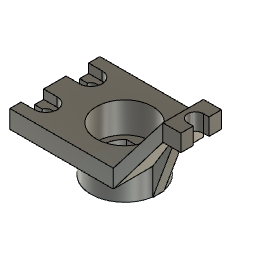
drawing_13 v1 (Autodesk Fusion 360 design; units mm, degrees)
Autodesk Fusion 360 part; units mm, degrees
sketch "Sketch1" plane through (0, 0, 0) normal (0, 0, 1) x (1, 0, 0)
  circle A0 centre (0, 0) radius 30
  constraint coincident A0.centre origin
extrude "Extrude1" add sketch "Sketch1" along normal blind 24 makes body 1
sketch "Sketch2" plane through (0, 0, 24) normal (0, 0, 1) x (-1, 0, 0)
  circle A0 centre (0, 0) radius 30
  line L0 (-30, 0) -> (-30, -40)
  line L1 (-30, -40) -> (-30, 0)
  line L2 (-30, 0) -> (-30, 40)
  line L3 (0, -40) -> (62, -40)
  line L4 (62, -40) -> (-30, -40)
  line L5 (-30, -40) -> (-30, 40)
  line L6 (-30, 40) -> (62, 40)
  line L7 (62, 40) -> (62, -40)
  constraint coincident A0.centre origin
  constraint coincident A0 L0.start
  constraint tangent A0 L1
  constraint perpendicular L0 L3
  constraint horizontal L4
  constraint vertical L5
  constraint horizontal L6
  constraint vertical L7
extrude "Extrude2" add sketch "Sketch2" along normal blind 16 contours A0 | L0 L1 L2 L3 L4 L5 L6 L7 bodies 1
sketch "Sketch3" plane through (0, 0, 40) normal (0, 0, 1) x (-1, 0, 0)
  line L0 (62, 40) -> (-30, 40)
  line L1 (-30, 40) -> (-30, -40)
  line L2 (-30, -40) -> (62, -40)
  line L3 (62, -40) -> (62, 40)
  line L4 (62, 0) -> (62, -20)
  line L5 (62, 0) -> (62, 20)
  line L6 (55.1235, 22) -> (62, 22)
  line L7 (62, 22) -> (62, 18)
  line L8 (62, 18) -> (55.1235, 18)
  line L9 (55.1235, -18) -> (62, -18)
  line L10 (62, -18) -> (62, -22)
  line L11 (62, -22) -> (55.1235, -22)
  arc A0 (59.798, -18) -> (59.798, -22) centre (50, -20) ccw
  arc A1 (55.1235, -18) -> (55.1235, -22) centre (50, -20) ccw
  arc A2 (59.798, 22) -> (59.798, 18) centre (50, 20) ccw
  arc A3 (55.1235, 22) -> (55.1235, 18) centre (50, 20) ccw
  point P0 (62, 0)
  constraint midpoint L3 P0
  constraint coincident P0 L4.start
  constraint parallel L3 L4
  constraint parallel L3 L5
  constraint concentric A0 A1
  constraint concentric A2 A3
  constraint horizontal L6
  constraint vertical L7
  constraint horizontal L8
  constraint coincident L3 L7.end
  constraint horizontal L9
  constraint vertical L10
  constraint horizontal L11
  constraint coincident L11 A0.end
  constraint coincident L9 A0.start
  constraint coincident L8 A2.end
  constraint coincident L6 A2.start
extrude "Extrude3" cut sketch "Sketch3" against normal blind 123 contours L3 L5 L6 L7 L8 A3 | L3 L4 L9 L10 L11 A1 bodies 1
sketch "Sketch4" plane through (0, 0, 40) normal (0, 0, 1) x (-1, 0, 0)
  line L0 (55.1235, 22) -> (62, 22)
  line L1 (62, 22) -> (62, 40)
  line L2 (62, 40) -> (-30, 40)
  line L3 (-30, 40) -> (-30, -40)
  line L4 (-30, -40) -> (62, -40)
  line L5 (62, -40) -> (62, -22)
  line L6 (62, -22) -> (55.1235, -22)
  arc A0 (55.1235, -18) -> (55.1235, -22) centre (50, -20) ccw
  line L7 (55.1235, -18) -> (62, -18)
  line L8 (62, -18) -> (62, 18)
  line L9 (62, 18) -> (55.1235, 18)
  arc A1 (55.1235, 22) -> (55.1235, 18) centre (50, 20) ccw
  circle A2 centre (50, -20) radius 10
  circle A3 centre (50, 20) radius 10
  line L10 (50, -30) -> (50, -10)
  line L11 (50, 30) -> (50, 10)
  line L12 (50, -30) -> (62, -30)
  line L13 (50, -10) -> (62, -10)
  line L14 (50, 10) -> (62, 10)
  line L15 (50, 30) -> (62, 30)
  dimension "d25" = 20
  dimension "d26" = 20
  constraint concentric A0 A2
  constraint concentric A1 A3
  constraint coincident A2 L10.start
  constraint coincident A2 L10.end
  constraint parallel L5 L10
  constraint coincident A3 L11.start
  constraint coincident A3 L11.end
  constraint parallel L10 L11
  constraint coincident L5 L12.end
  constraint tangent A2 L12
  constraint perpendicular L5 L12
  constraint coincident L8 L13.end
  constraint tangent A2 L13
  constraint coincident L8 L14.end
  constraint tangent A3 L14
  constraint perpendicular L8 L14
  constraint coincident L1 L15.end
  constraint tangent A3 L15
  measures "d25" diameter of A2
  measures "d26" diameter of A3
extrude "Extrude4" cut sketch "Sketch4" against normal blind 8 contours L0 A1 A3 L11 | L0 L1 A3 L15 | A1 A3 L11 | L9 A1 A3 L11 | L8 L9 A3 L14 | L7 L8 A2 L13 | A0 A2 L10 | A0 L7 A2 L10 | L6 A0 A2 L10 | L5 L6 A2 L12 bodies 1
sketch "Sketch5" plane through (0, -40, 0) normal (0, -1, 0) x (1, 0, 0)
  line L0 (-62, 24) -> (30, 24)
  line L1 (30, 24) -> (30, 40)
  line L2 (30, 40) -> (-62, 40)
  line L3 (-62, 40) -> (-62, 24)
  line L4 (52, 55) -> (52, 70)
  line L5 (52, 70) -> (52, 55)
  line L6 (30, 40) -> (52, 70)
  line L7 (30, 24) -> (52, 55)
  constraint coincident L1.end L2.start
  constraint parallel L4 L5
  constraint coincident L0.end L1.start
sketch "Sketch6" plane through (0, 40, 0) normal (0, 1, 0) x (-1, 0, 0)
  line L0 (-30, 24) -> (62, 24)
  line L1 (62, 24) -> (62, 40)
  line L2 (62, 40) -> (-30, 40)
  line L3 (-30, 40) -> (-30, 24)
  line L4 (62, 24) -> (-52, 24)
  line L5 (-52, 24) -> (-52, 26)
  line L6 (-52, 26) -> (-30, 26)
  line L7 (-30, 24) -> (-30, 26)
  dimension "d34" = 114
  dimension "d35" = 2
  constraint coincident L0.end L1.start
  constraint perpendicular L1 L4
  constraint perpendicular L4 L5
  constraint coincident L3 L6.end
  constraint perpendicular L3 L6
  constraint coincident L0.start L3.end
  measures "d34" distance of L0.end L4.end
  measures "d35" distance of L4.end L5.end
ref_plane "WorkPlane3" through (0, 0, 75) normal (0, 0, -1) x (-1, 0, 0)
sketch "Sketch23" plane through (0, 0, 75) normal (0, 0, -1) x (1, 0, 0)
  line L0 (-62, -30) -> (-50, -30) construction
  arc A0 (-50, -30) -> (-50, -10) centre (-50, -20) ccw construction
  line L1 (-50, -10) -> (-62, -10) construction
  line L2 (-62, -10) -> (-62, 10) construction
  line L3 (-62, 10) -> (-50, 10) construction
  arc A1 (-50, 10) -> (-50, 30) centre (-50, 20) ccw construction
  line L4 (-50, 30) -> (-62, 30) construction
  line L5 (-62, 30) -> (-62, 40) construction
  line L6 (-62, 40) -> (30, 40) construction
  line L7 (30, 40) -> (30, -40) construction
  line L8 (30, -40) -> (-62, -40) construction
  line L9 (-62, -40) -> (-62, -30) construction
  line L10 (-62, 0) -> (68, 0) construction
  line L11 (68, 0) -> (52, 0) construction
  line L12 (52, 0) -> (52, -18) construction
  line L13 (52, -18) -> (52, 18) construction
  line L14 (68, -18) -> (52, -18)
  line L15 (52, -18) -> (52, 18)
  line L16 (52, 18) -> (68, 18)
  line L17 (68, 18) -> (68, -18)
  line L18 (68, -18) -> (52, 18) construction
  line L19 (52, -18) -> (68, 18) construction
  circle A2 centre (0, 0) radius 30 construction
  line L20 (0, 0) -> (63, 0) construction
  line L21 (63, -7) -> (77.3975, -7)
  arc A3 (77.3975, -7) -> (77.3975, 7) centre (77.3975, 0) ccw
  line L22 (77.3975, 7) -> (63, 7)
  arc A4 (63, 7) -> (63, -7) centre (63, 0) ccw
  line L23 (63, 0) -> (77.3975, 0) construction
  point P0 (60, 0)
  dimension "d68" = 130
  dimension "d69" = 16
  dimension "d72" = 16
  dimension "d73" = 36
  dimension "d74" = 63
  dimension "d75" = 14
  constraint midpoint L2 L10.start
  constraint perpendicular L2 L10
  constraint coincident L10 L11.end
  constraint perpendicular L11 L12
  constraint perpendicular L10 L13
  constraint horizontal L14
  constraint perpendicular L14 L15
  constraint parallel L14 L16
  constraint parallel L15 L17
  constraint coincident L18 P0
  constraint coincident L19 P0
  constraint midpoint L11 P0
  constraint coincident A2.centre L20.start
  constraint parallel L10 L20
  constraint tangent L21 A3
  constraint tangent A3 L22
  constraint parallel L21 L22
  constraint tangent L22 A4
  constraint tangent L21 A4
  constraint perpendicular L17 L23
  constraint coincident L20.end A4.centre
  measures "d68" distance of L10.start L10.end
  measures "d69" distance of L10.end L11.end
  measures "d72" distance of L13.end L16.end
  measures "d73" distance of L12.end L13.end
  measures "d74" distance of A2.centre L20.end
  measures "d75" diameter of A3
extrude "Extrude15" add sketch "Sketch23" along normal blind 15 separate body contours L14 L15 L16 L17 L21 L22 A4 makes body 2
loft "Loft1" add section 1 face at (52, 6, 70) section 2 face at (30, 0, 34.6667) on bodies 1 2 bodies 2 1
sketch "Sketch24" plane through (0, 0, 0) normal (0, 1, 0) x (1, 0, 0)
  line L0 (52, -75) -> (30, -40)
  line L1 (52, -60) -> (30, -24)
  line L2 (-62, -40) -> (30, -40)
  line L3 (-62, -24) -> (-62, -40)
  line L4 (-30, -24) -> (-62, -24)
  line L5 (-30, 0) -> (30, 0)
  line L6 (52, -75) -> (68, -75)
  line L7 (68, -60) -> (52, -60)
  line L8 (68, -75) -> (68, -60)
  line L9 (-30, 0) -> (-30, -24)
  line L10 (30, 0) -> (30, -24)
  line L11 (30, 0) -> (52, -60)
  constraint coincident L5.end L10.start
  constraint coincident L1.start L7.end
extrude "Extrude16" add sketch "Sketch24" along normal mid plane 10 separate body contours L1 L10 L11 makes body 3
sketch "Sketch25" plane through (0, 0, 0) normal (0, 0, -1) x (1, 0, 0)
  circle A0 centre (0, 0) radius 30
sketch "Sketch14" plane through (0, 0, 40) normal (0, 0, 1) x (-1, 0, 0)
  line L0 (62, -30) -> (50, -30)
  arc A0 (50, -10) -> (50, -30) centre (50, -20) ccw
  line L1 (50, -10) -> (62, -10)
  line L2 (62, -10) -> (62, 10)
  line L3 (62, 10) -> (50, 10)
  arc A1 (50, 30) -> (50, 10) centre (50, 20) ccw
  line L4 (50, 30) -> (62, 30)
  line L5 (62, 30) -> (62, 40)
  line L6 (62, 40) -> (-30, 40)
  line L7 (-30, -40) -> (62, -40)
  circle A2 centre (0, 0) radius 25
  line L8 (-30, 40) -> (-30, -40)
  line L9 (62, -40) -> (62, -30)
  dimension "d53" = 50
  constraint coincident A2.centre origin
  measures "d53" diameter of A2
extrude "Extrude12" cut sketch "Sketch14" against normal blind 27 contours A2 bodies 2
sketch "Sketch15" plane through (0, 0, 0) normal (0, 0, -1) x (1, 0, 0)
  circle A0 centre (0, 0) radius 30
  circle A1 centre (0, 0) radius 11
  dimension "d56" = 22
  constraint coincident A0.centre A1.centre
  measures "d56" diameter of A1
sketch "Sketch16" plane through (0, 0, 13) normal (0, 0, 1) x (-1, 0, 0)
  circle A0 centre (0, 0) radius 25
  line L0 (0, 0) -> (0, -15)
  line L1 (0, -15) -> (0, 0)
  line L2 (0, 0) -> (0, 15)
  line L3 (0, -15) -> (-13.2288, -15)
  line L4 (13.2288, -15) -> (0, -15)
  line L5 (0, 15) -> (-13.2288, 15)
  line L6 (0, 15) -> (13.2288, 15)
  arc A1 (13.2288, -15) -> (13.2288, 15) centre (0, 0) ccw
  arc A2 (-13.2288, 15) -> (-13.2288, -15) centre (0, 0) ccw
  constraint coincident A0.centre L0.start
  constraint vertical L0
  constraint parallel L0 L2
  constraint perpendicular L1 L3
  constraint perpendicular L0 L4
  constraint coincident L5.end A1
  constraint perpendicular L2 L5
  constraint perpendicular L2 L6
  constraint concentric A1 A2
extrude "Extrude14" cut sketch "Sketch16" against normal blind 12 contours L0 L1 L2 L4 L6 A1 | L0 L1 L2 L3 L5 A2 bodies 2
extrude "Extrude13" cut sketch "Sketch15" against normal blind 45 contours A1 bodies 2
